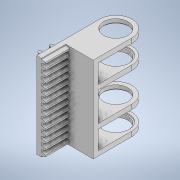
# Autodesk Inventor part: Wechsel_Schiebeteil
Saved by Autodesk Inventor 2021 (Build 250183000, 183)
## iProperties
Created: 2021-01-25
Part Number: Wechsel_Schiebeteil
Material: Generisch
Document SubType Name: Modeling
Designer: Jaro Machnow
Density: 1 g/cm^3
Appearance: Vorgabe
Author: Jaro Machnow
Autodesk Inventor part; units mm, degrees
sketch "Skizze1" plane through (0, 0, 0) normal (0, 1, 0) x (-1, 0, 0)
  circle A0 centre (0, 0) radius 7.5
  arc A1 (-10, 0) -> (10, 0) centre (0, 0) ccw
  line L0 (7.5, 0) -> (-7.5, 0)
  line L1 (-10, 0) -> (-10, 21)
  line L2 (-10, 21) -> (10, 21)
  line L3 (10, 21) -> (10, 0)
  dimension "d0" = 15
  dimension "d1" = 20
  dimension "d2" = 21
  constraints: 8 end point, 4 point on circle, 2 centre point, 2 coincident, 2 parallel, 1 horizontal, 1 perpendicular
  measures "d0" diameter of A0
  measures "d1" diameter of A1
  measures "d2" distance of L1.start L1.end
extrude "Extrusion1" add sketch "Skizze1" along normal blind 3
sketch "Skizze2" plane through (0, 3, 0) normal (0, 1, 0) x (1, 0, 0)
  circle A0 centre (0, 0) radius 8.25
  dimension "d5" = 16.5
  constraints: 1 centre point, 1 coincident
  measures "d5" diameter of A0
extrude "Extrusion2" cut sketch "Skizze2" against normal blind 0.8
ref_plane "Arbeitsebene2" through (10, 14.5, 21) normal (0, 1, 0) x (1, 0, 0)
ref_plane "Arbeitsebene1" through (10, 3, 21) normal (0, 1, 0) x (1, 0, 0)
sketch "Skizze3" plane through (10, 14.5, 21) normal (0, 1, 0) x (1, 0, 0)
  circle A0 centre (-10, 21) radius 7.5
  arc A1 (0, 21) -> (-20, 21) centre (-10, 21) ccw projected
  arc A2 (0, 21) -> (-20, 21) centre (-10, 21) ccw
  line L0 (-20, 21) -> (-20, 0) projected
  line L1 (-20, 0) -> (0, 0) projected
  line L2 (-17.5, 21) -> (-2.5, 21)
  line L3 (0, 21) -> (0, 0)
  line L4 (0, 0) -> (-20, 0)
  line L5 (-20, 0) -> (-20, 21)
  dimension "d9" = 15
  constraints: 8 end point, 4 point on circle, 2 centre point, 2 coincident, 2 parallel, 1 horizontal, 1 perpendicular
  measures "d9" diameter of A0
extrude "Extrusion3" add sketch "Skizze3" along normal blind 3
sketch "Skizze4" plane through (10, 14.5, 21) normal (0, 1, 0) x (1, 0, 0)
  circle A0 centre (-10, 21) radius 8.25
  dimension "d12" = 16.5
  constraints: 1 centre point, 1 coincident
  measures "d12" diameter of A0
extrude "Extrusion4" cut sketch "Skizze4" along normal blind 0.8
ref_plane "Arbeitsebene3" through (0, -9, 0) normal (0, 1, 0) x (-1, 0, 0)
sketch "Skizze5" plane through (0, -9, 0) normal (0, 1, 0) x (-1, 0, 0)
  point P0 (0, 0)
mirror "Spiegeln1" about plane through (0, -9, 0) normal (0, 1, 0) of "Extrusion3", "Extrusion1"
sketch "Skizze6" plane through (0, -21, 0) normal (0, -1, 0) x (1, 0, 0)
  circle A0 centre (0, 0) radius 8.25
  dimension "d16" = 16.5
  constraints: 1 centre point, 1 coincident
  measures "d16" diameter of A0
extrude "Extrusion5" cut sketch "Skizze6" against normal blind 0.8
sketch "Skizze7" plane through (0, -32.5, 0) normal (0, 1, 0) x (1, 0, 0)
  circle A0 centre (0, 0) radius 8.25
  dimension "d19" = 16.5
  constraints: 1 centre point, 1 coincident
  measures "d19" diameter of A0
extrude "Extrusion6" cut sketch "Skizze7" against normal blind 0.8
ref_plane "Arbeitsebene4" through (10, 17.5, 21) normal (0, 0, 1) x (1, 0, 0)
sketch "Skizze8" plane through (10, 17.5, 21) normal (0, 0, 1) x (1, 0, 0)
  line L0 (0, 0) -> (-20, 0) projected
  line L1 (0, -53) -> (-20, -53) projected
  line L2 (0, 0) -> (-20, 0)
  line L3 (-20, 0) -> (-20, -53)
  line L4 (-20, -53) -> (0, -53)
  line L5 (0, -53) -> (0, 0)
  point P0 (-10, -17.5)
  constraints: 8 end point, 2 parallel, 1 horizontal, 1 perpendicular
extrude "Extrusion7" add sketch "Skizze8" along normal blind 3
sketch "Skizze9" plane through (10, 17.5, 24) normal (0, 0, 1) x (1, 0, 0)
  arc A0 (-14.6847, -1.0523) -> (-17, -0.5195) centre (-17.407, -7.5844) ccw
  arc A1 (-14.6847, -1.942) -> (-14.6847, -1.0523) centre (-23.1731, -1.4972) ccw
  arc A2 (-17, -2.4749) -> (-14.6847, -1.942) centre (-17.407, 4.59) ccw
  line L0 (-17, -0.5195) -> (-17, 0) construction
  line L1 (-20, -3) -> (-20, 0) projected
  line L2 (0, -53) -> (-20, -53) projected
  line L3 (-20, 0) -> (-17, 0)
  line L4 (-17, -53) -> (-20, -53)
  line L5 (-20, -53) -> (-20, 0)
  arc A3 (-17, -6.0354) -> (-14.6847, -5.5025) centre (-17.407, 1.0295) ccw
  arc A4 (-14.6847, -5.5025) -> (-14.6847, -4.6128) centre (-23.1731, -5.0577) ccw
  arc A5 (-14.6847, -4.6128) -> (-17, -4.0799) centre (-17.407, -11.1449) ccw
  arc A6 (-17, -9.5958) -> (-14.6847, -9.063) centre (-17.407, -2.5309) ccw
  arc A7 (-14.6847, -9.063) -> (-14.6847, -8.1733) centre (-23.1731, -8.6181) ccw
  arc A8 (-14.6847, -8.1733) -> (-17, -7.6404) centre (-17.407, -14.7053) ccw
  arc A9 (-17, -13.1563) -> (-14.6847, -12.6234) centre (-17.407, -6.0914) ccw
  arc A10 (-14.6847, -12.6234) -> (-14.6847, -11.7337) centre (-23.1731, -12.1786) ccw
  arc A11 (-14.6847, -11.7337) -> (-17, -11.2009) centre (-17.407, -18.2658) ccw
  arc A12 (-17, -16.7168) -> (-14.6847, -16.1839) centre (-17.407, -9.6519) ccw
  arc A13 (-14.6847, -16.1839) -> (-14.6847, -15.2942) centre (-23.1731, -15.7391) ccw
  arc A14 (-14.6847, -15.2942) -> (-17, -14.7614) centre (-17.407, -21.8263) ccw
  arc A15 (-17, -20.2773) -> (-14.6847, -19.7444) centre (-17.407, -13.2123) ccw
  arc A16 (-14.6847, -19.7444) -> (-14.6847, -18.8547) centre (-23.1731, -19.2995) ccw
  arc A17 (-14.6847, -18.8547) -> (-17, -18.3218) centre (-17.407, -25.3867) ccw
  arc A18 (-17, -23.8377) -> (-14.6847, -23.3049) centre (-17.407, -16.7728) ccw
  arc A19 (-14.6847, -23.3049) -> (-14.6847, -22.4152) centre (-23.1731, -22.86) ccw
  arc A20 (-14.6847, -22.4152) -> (-17, -21.8823) centre (-17.407, -28.9472) ccw
  arc A21 (-17, -27.3982) -> (-14.6847, -26.8653) centre (-17.407, -20.3333) ccw
  arc A22 (-14.6847, -26.8653) -> (-14.6847, -25.9756) centre (-23.1731, -26.4205) ccw
  arc A23 (-14.6847, -25.9756) -> (-17, -25.4428) centre (-17.407, -32.5077) ccw
  arc A24 (-17, -30.9587) -> (-14.6847, -30.4258) centre (-17.407, -23.8938) ccw
  arc A25 (-14.6847, -30.4258) -> (-14.6847, -29.5361) centre (-23.1731, -29.981) ccw
  arc A26 (-14.6847, -29.5361) -> (-17, -29.0032) centre (-17.407, -36.0682) ccw
  arc A27 (-17, -34.5191) -> (-14.6847, -33.9863) centre (-17.407, -27.4542) ccw
  arc A28 (-14.6847, -33.9863) -> (-14.6847, -33.0966) centre (-23.1731, -33.5414) ccw
  arc A29 (-14.6847, -33.0966) -> (-17, -32.5637) centre (-17.407, -39.6286) ccw
  arc A30 (-17, -38.0796) -> (-14.6847, -37.5468) centre (-17.407, -31.0147) ccw
  arc A31 (-14.6847, -37.5468) -> (-14.6847, -36.657) centre (-23.1731, -37.1019) ccw
  arc A32 (-14.6847, -36.657) -> (-17, -36.1242) centre (-17.407, -43.1891) ccw
  arc A33 (-17, -41.6401) -> (-14.6847, -41.1072) centre (-17.407, -34.5752) ccw
  arc A34 (-14.6847, -41.1072) -> (-14.6847, -40.2175) centre (-23.1731, -40.6624) ccw
  arc A35 (-14.6847, -40.2175) -> (-17, -39.6847) centre (-17.407, -46.7496) ccw
  arc A36 (-17, -45.2006) -> (-14.6847, -44.6677) centre (-17.407, -38.1356) ccw
  arc A37 (-14.6847, -44.6677) -> (-14.6847, -43.778) centre (-23.1731, -44.2228) ccw
  arc A38 (-14.6847, -43.778) -> (-17, -43.2451) centre (-17.407, -50.31) ccw
  arc A39 (-17, -48.761) -> (-14.6847, -48.2282) centre (-17.407, -41.6961) ccw
  arc A40 (-14.6847, -48.2282) -> (-14.6847, -47.3385) centre (-23.1731, -47.7833) ccw
  arc A41 (-14.6847, -47.3385) -> (-17, -46.8056) centre (-17.407, -53.8705) ccw
  arc A42 (-17, -52.3215) -> (-14.6847, -51.7886) centre (-17.407, -45.2566) ccw
  arc A43 (-14.6847, -51.7886) -> (-14.6847, -50.8989) centre (-23.1731, -51.3438) ccw
  arc A44 (-14.6847, -50.8989) -> (-17, -50.3661) centre (-17.407, -57.431) ccw
  line L6 (-17, 0) -> (-17, -0.5195)
  line L7 (-17, -2.4749) -> (-17, -4.0799)
  line L8 (-17, -6.0354) -> (-17, -7.6404)
  line L9 (-17, -9.5958) -> (-17, -11.2009)
  line L10 (-17, -13.1563) -> (-17, -14.7614)
  line L11 (-17, -16.7168) -> (-17, -18.3218)
  line L12 (-17, -20.2773) -> (-17, -21.8823)
  line L13 (-17, -23.8377) -> (-17, -25.4428)
  line L14 (-17, -27.3982) -> (-17, -29.0032)
  line L15 (-17, -30.9587) -> (-17, -32.5637)
  line L16 (-17, -34.5191) -> (-17, -36.1242)
  line L17 (-17, -38.0796) -> (-17, -39.6847)
  line L18 (-17, -41.6401) -> (-17, -43.2451)
  line L19 (-17, -45.2006) -> (-17, -46.8056)
  line L20 (-17, -48.761) -> (-17, -50.3661)
  line L21 (-17, -52.3215) -> (-17, -53)
  point P0 (-10, -17.5)
  dimension "d30" = 10
  dimension "d24" = 3
  dimension "d27" = 3.5605
  constraints: 90 point on circle, 45 centre point, 40 end point, 17 parallel, 16 perpendicular, 1 horizontal, 1 point on line
  measures "d24" distance of L4.start L4.end
  measures "d27" distance of A2.centre A3.centre
extrude "Extrusion8" add sketch "Skizze9" along normal blind 15
sketch "Skizze10" plane through (-10, -18, 21) normal (-1, 0, 0) x (0, 0, 1)
  line L0 (15, -17.5) -> (13, -17.5)
  line L1 (13, -17.5) -> (13, 35.5)
  line L2 (13, 35.5) -> (15, 35.5)
  line L3 (15, 35.5) -> (15, -17.5)
  line L4 (8, -17.5) -> (6, -17.5)
  line L5 (6, -17.5) -> (6, 35.5)
  line L6 (6, 35.5) -> (8, 35.5)
  line L7 (8, 35.5) -> (8, -17.5)
  line L8 (10.5, -63.5631) -> (10.5, -1.5631) construction
  line L9 (18, 35.5) -> (18, -17.5) projected
  line L10 (3, 34.4477) -> (18, 34.4477) projected
  line L11 (-21, 35.5) -> (18, 35.5) projected
  line L12 (-21, -17.5) -> (18, -17.5) projected
  point P0 (-21, 18)
  point P1 (15, 34.4477)
  point P2 (13, 34.4477)
  point P3 (8, 34.4477)
  point P4 (6, 34.4477)
  dimension "d34" = 2
  dimension "d36" = 5
  dimension "d37" = 7.5
  constraints: 18 end point, 4 parallel, 4 point on line, 2 horizontal, 2 perpendicular, 2 other
  measures "d34" distance of L1.end L2.end
  measures "d36" distance between parallel lines of L1 L7
  measures "d37" distance between parallel lines of L9 L8
extrude "Extrusion9" add sketch "Skizze10" along normal blind 3 contours L0 L1 L10 L3 | L4 L5 L10 L7
fillet "Rundung1" radius 1 4 edges at (-13, -9.5262, 27) (-13, -9.5262, 29) (-13, -9.5262, 34) (-13, -9.5262, 36)
